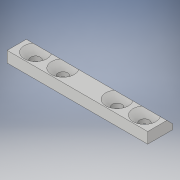
# Autodesk Inventor part: topSpacer
Saved by Autodesk Inventor 2017 (Build 210142000, 142)
## iProperties
Created: 2022-11-19
Part Number: topSpacer
Material: Generic
Document SubType Name: Modeling
Designer: khonsu
Density: 1 g/cm^3
Appearance: Default
Author: khonsu
Autodesk Inventor part; units mm, degrees
ref_plane "YZ Plane" through (0, 0, 0) normal (1, 0, 0) x (0, 1, 0)
ref_plane "XZ Plane" through (0, 0, 0) normal (0, 1, 0) x (-1, 0, 0)
ref_plane "XY Plane" through (0, 0, 0) normal (0, 0, 1) x (1, 0, 0)
sketch "Sketch1" plane through (0, 0, 0) normal (0, 1, 0) x (-1, 0, 0)
  line L0 (0, 0) -> (-20.772, 0)
  line L1 (-20.772, 0) -> (-20.772, -9.19)
  line L2 (-20.772, -9.19) -> (0, -9.19)
  line L3 (0, -9.19) -> (0, 0)
  line L4 (-20.772, -9.19) -> (-30.572, -9.19)
  line L5 (-30.572, -9.19) -> (-30.572, 0)
  line L6 (-30.572, 0) -> (-20.772, 0)
  line L7 (-20.772, 0) -> (-20.772, -9.19)
  line L8 (-30.572, -9.19) -> (-51.344, -9.19)
  line L9 (-51.344, -9.19) -> (-51.344, 0)
  line L10 (-51.344, 0) -> (-30.572, 0)
  line L11 (-30.572, 0) -> (-30.572, -9.19)
  circle A0 centre (-5.772, -4.595) radius 1.75
  circle A1 centre (-15.772, -4.595) radius 1.75
  circle A2 centre (-35.572, -4.595) radius 1.75
  circle A3 centre (-45.572, -4.595) radius 1.75
  dimension "d0" = 20.772
  dimension "d1" = 9.19
  dimension "d2" = 9.8
  dimension "d3" = 9.19
  dimension "d4" = 20.772
  dimension "d5" = 9.19
  dimension "d6" = 3.5
  dimension "d7" = 3.5
  dimension "d8" = 3.5
  dimension "d9" = 3.5
  dimension "d10" = 5.772
  dimension "d11" = 10
  dimension "d12" = 5.772
  dimension "d13" = 10
  constraints: 24 end point, 6 parallel, 4 centre point, 3 horizontal, 3 perpendicular
  measures "d0" distance of L2.end L1.end
  measures "d1" distance of L1.end L0.end
  measures "d2" distance of L5.end L6.end
  measures "d3" distance of L4.end L5.end
  measures "d4" distance of L9.end L10.end
  measures "d5" distance of L8.end L9.end
  measures "d6" diameter of A0
  measures "d7" diameter of A1
  measures "d8" diameter of A2
  measures "d9" diameter of A3
  measures "d10" distance from line of L3 A0.centre
  measures "d11" distance of A0.centre A1.centre
  measures "d12" distance from line of L9 A3.centre
  measures "d13" distance of A3.centre A2.centre
extrude "Extrusion1" add sketch "Sketch1" along normal blind 4
chamfer "Chamfer1" distance 2.1825 angle 45 1 edges at (25.672, 4, -9.19)
chamfer "Chamfer2" distance 2.4 angle 45 4 edges at (7.522, 4, -4.595) (17.522, 4, -4.595) (37.322, 4, -4.595) (47.322, 4, -4.595)
equation "\"d12\" = d10"
equation "\"d13\" = d11"
body "Solid1"
